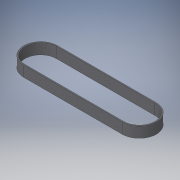
# Autodesk Inventor part: 5.5belt
Saved by Autodesk Inventor 2018 (Build 220112000, 112)
## iProperties
Created: 2019-01-10
Part Number: 5.5belt
Material: Generic
Document SubType Name: Modeling
Designer: snipe
Density: 1 g/cm^3
Appearance: Iron - Cast
Author: snipe
Autodesk Inventor part; units mm, degrees
ref_plane "YZ Plane" through (0, 0, 0) normal (1, 0, 0) x (0, 1, 0)
ref_plane "XZ Plane" through (0, 0, 0) normal (0, 1, 0) x (-1, 0, 0)
ref_plane "XY Plane" through (0, 0, 0) normal (0, 0, 1) x (1, 0, 0)
sketch "Sketch1" plane through (0, 0, 0) normal (0, 1, 0) x (-1, 0, 0)
  line L0 (0, -33.6) -> (0, 33.6) projected
  line L1 (-140.8201, 0) -> (186.8327, 0) projected
  line L2 (186.8327, 0) -> (-140.8201, 0) projected
  line L3 (0, -33.6) -> (0, 33.6) projected
  line L4 (70.0126, 0) -> (-70.0126, 0) construction
  line L5 (70.0126, 24) -> (-70.0126, 24)
  line L6 (-70.0126, -24) -> (70.0126, -24)
  arc A0 (70.0126, -24) -> (70.0126, 24) centre (70.0126, 0) ccw
  arc A1 (-70.0126, 24) -> (-70.0126, -24) centre (-70.0126, 0) ccw
  line L7 (0, 0) -> (140.0251, 0) construction
  line L8 (70.0126, -22.225) -> (-70.0126, -22.225)
  arc A2 (-70.0126, 22.225) -> (-70.0126, -22.225) centre (-70.0126, 0) ccw
  line L9 (-70.0126, 22.225) -> (70.0126, 22.225)
  arc A3 (70.0126, -22.225) -> (70.0126, 22.225) centre (70.0126, 0) ccw
  dimension "d0" = 70.0126
  dimension "d1" = 180
  dimension "d2" = 48
  dimension "d3" = 1.775
  constraints: 14 end point, 8 point on circle, 4 centre point, 4 tangent, 2 parallel, 1 collinear, 1 horizontal, 1 midpoint, 1 perpendicular, 3 other
  measures "d0" distance of L7.start L4.end
  measures "d1" angle of L4 L7
  measures "d2" diameter of A1
  measures "d3" distance between parallel lines of L6 L8
extrude "Extrusion1" add sketch "Sketch1" along normal blind 15 contours L6 A1 L1 A2 L8 L0 | L0 L8 A3 L1 A0 L6 | A1 L5 L0 L9 A2 L1 | L1 A3 L9 L0 L5 A0
body "Solid1"
